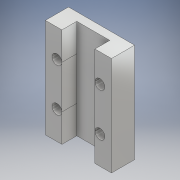
# Autodesk Inventor part: slider_b7p5x20_30_sa
Saved by Autodesk Inventor 2018 (Build 220112000, 112)
## iProperties
Created: 2018-02-22
Part Number: slider_b7p5x20_30_sa
Material: アルミニウム 6061-AHC
Document SubType Name: Modeling
Designer: shun
Density: 2.7 g/cm^3
Appearance: アルミニウム - ダーク
Author: shun
Autodesk Inventor part; units mm, degrees
ref_plane "YZ Plane" through (0, 0, 0) normal (1, 0, 0) x (0, 1, 0)
ref_plane "XZ Plane" through (0, 0, 0) normal (0, 1, 0) x (-1, 0, 0)
ref_plane "XY Plane" through (0, 0, 0) normal (0, 0, 1) x (1, 0, 0)
sketch "スケッチ1" plane through (0, 0, 0) normal (0, 0, 1) x (1, 0, 0)
  line L0 (-10, -7) -> (-5, -7)
  line L1 (10, -7) -> (10, 0)
  line L2 (10, 0) -> (-10, 0)
  line L3 (-10, 0) -> (-10, -7)
  line L4 (-10, -7) -> (10, 0) construction
  line L5 (10, -7) -> (-10, 0) construction
  line L6 (-5, -2.5) -> (5, -2.5)
  line L7 (5, -2.5) -> (5, -7)
  line L8 (-5, -7) -> (-5, -2.5)
  line L9 (-5, -2.5) -> (5, -7) construction
  line L10 (5, -2.5) -> (-5, -7) construction
  line L11 (5, -7) -> (10, -7)
  point P0 (0, 0)
  point P1 (0, -3.5)
  point P2 (0, -4.75)
  dimension "d0" = 20
  dimension "d1" = 7
  dimension "d2" = 10
  dimension "d3" = 4.5
  constraints: 24 end point, 4 midpoint, 4 parallel, 3 horizontal, 3 perpendicular
  measures "d0" distance of L2.end L1.end
  measures "d1" distance of L1.start L1.end
  measures "d2" distance of L7.end L0.end
  measures "d3" distance of L6.end L7.end
extrude "押し出し1" add sketch "スケッチ1" along normal blind 30
sketch "スケッチ2" plane through (-10, 0, 0) normal (0, 1, 0) x (1, 0, 0)
  line L0 (0, 0) -> (0, -30) projected
  line L1 (20, 0) -> (0, 0) projected
  line L2 (20, -30) -> (0, -30) projected
  line L3 (20, 0) -> (20, -30) projected
  point P0 (10, 0)
  point P1 (3.5, -8.5)
  point P2 (3.5, -21.5)
  point P3 (16.5, -21.5)
  point P4 (16.5, -8.5)
  dimension "d6" = 3.5
  dimension "d7" = 3.5
  dimension "d8" = 8.5
  dimension "d9" = 8.5
  dimension "d10" = 3.5
  dimension "d11" = 3.5
  dimension "d12" = 8.5
  dimension "d13" = 8.5
  measures "d6" distance from line of L0 point (3.5, -8.5)
  measures "d7" distance from line of L0 point (3.5, -21.5)
  measures "d8" distance from line of L1 point (3.5, -8.5)
  measures "d9" distance from line of L2 point (3.5, -21.5)
  measures "d10" distance from line of L3 point (16.5, -8.5)
  measures "d11" distance from line of L3 point (16.5, -21.5)
  measures "d12" distance from line of L1 point (16.5, -8.5)
  measures "d13" distance from line of L2 point (16.5, -21.5)
hole "穴1" at (-6.5, 0, 8.5) at (-6.5, 0, 21.5) at (6.5, 0, 21.5) at (6.5, 0, 8.5) direction (0, -1, 0) diameter 3 end through all
equation "\"d7\" = d6"
equation "\"d9\" = d8"
equation "\"d10\" = d6"
equation "\"d11\" = d6"
equation "\"d12\" = d8"
equation "\"d13\" = d8"
